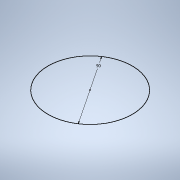
# Autodesk Inventor part: Container_Design1
Saved by Autodesk Inventor 2022 (Build 260153070, 153G)
## iProperties
Created: 2022-04-01
Part Number: Container_Design1
Material: Generic
Document SubType Name: Modeling
Designer: a laptop
Density: 1 g/cm^3
Appearance: Default
Author: a laptop
Autodesk Inventor part; units mm, degrees
ref_plane "YZ Plane" through (0, 0, 0) normal (1, 0, 0) x (0, 1, 0)
ref_plane "XZ Plane" through (0, 0, 0) normal (0, 1, 0) x (-1, 0, 0)
ref_plane "XY Plane" through (0, 0, 0) normal (0, 0, 1) x (1, 0, 0)
sketch "Sketch2" plane through (0, 0, 0) normal (0, 1, 0) x (-1, 0, 0)
  ellipse E0 centre (0, 0) end of major axis (0, -27.831227) minor radius 45.991949
  line L0 (-45.991949, 13.746993) -> (-45.991949, 0)
  arc A0 (8.739669, 27.324115) -> (-38.789406, 23.347735) centre (-5.219918, -91.86116) ccw
  arc A1 (-38.789406, 23.347735) -> (-45.991949, 13.746993) centre (-35.991949, 13.746993) ccw
  point P0 (-45.991949, 21)
  dimension "d9" = 10
  dimension "d10" = 120
  dimension "d11" = 21
  constraints: 5 point on circle, 2 centre point, 2 end point, 2 tangent, 2 vertical, 1 coincident, 1 point on line, 5 other
  measures "d9" radius of A1
  measures "d10" radius of A0
  measures "d11" vertical distance of point (-45.992, 21) point (0, 0)
extrude "Extrusion4" add sketch "Sketch2" along normal blind 300
shell "Shell1" thickness 2 outward yes removed faces 1 at (0.597516, 300, -9.012044)
fillet "Fillet1" radius 5 4 edges at (15.3912, -2, 29.7141) (45.591, -2, 20.9483) (47.9919, -2, 6.8735) (-25.9313, -2, -25.1431)
body "Solid2"
